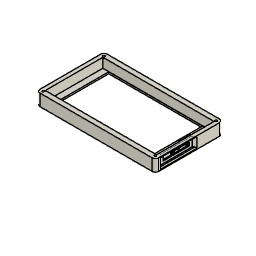
Display Mount - TFT70V30 SD Access Cover (Autodesk Fusion 360 design; units mm, degrees)
Autodesk Fusion 360 part; units mm, degrees
sketch "Sketch1" plane through (0, 0, -12) normal (0, 0, -1) x (1, 0, 0)
  line L0 (-106, 54.1) -> (-106, -54.1)
  line L1 (-100, -60.1) -> (100, -60.1)
  line L2 (106, -54.1) -> (106, 54.1)
  line L3 (100, 60.1) -> (-100, 60.1)
  arc A0 (4.9335, 51.1) -> (-4.9335, 51.1) centre (0, 51.9125) ccw
  arc A1 (86.5835, 51.1) -> (76.7165, 51.1) centre (81.65, 51.9125) ccw
  line L4 (86.5835, 51.1) -> (99, 51.1)
  line L5 (99, 51.1) -> (99, -51.1)
  line L6 (99, -51.1) -> (86.5835, -51.1)
  arc A2 (76.7165, -51.1) -> (86.5835, -51.1) centre (81.65, -51.9125) ccw
  arc A3 (-4.9335, -51.1) -> (4.9335, -51.1) centre (0, -51.9125) ccw
  arc A4 (-86.5835, -51.1) -> (-76.7165, -51.1) centre (-81.65, -51.9125) ccw
  line L7 (-86.5835, -51.1) -> (-99, -51.1)
  line L8 (-99, -51.1) -> (-99, 51.1)
  line L9 (-99, 51.1) -> (-86.5835, 51.1)
  arc A5 (-76.7165, 51.1) -> (-86.5835, 51.1) centre (-81.65, 51.9125) ccw
  circle A6 centre (-100, -54.1) radius 2.3
  circle A7 centre (100, -54.1) radius 2.3
  circle A8 centre (-100, 54.1) radius 2.3
  circle A9 centre (100, 54.1) radius 2.3
  arc A10 (106, 54.1) -> (100, 60.1) centre (100, 54.1) ccw
  arc A11 (-100, 60.1) -> (-106, 54.1) centre (-100, 54.1) ccw
  arc A12 (-106, -54.1) -> (-100, -60.1) centre (-100, -54.1) ccw
  arc A13 (100, -60.1) -> (106, -54.1) centre (100, -54.1) ccw
  line L10 (5.2198, 51.35) -> (76.4302, 51.35)
  line L11 (-5.2198, -51.35) -> (-76.4302, -51.35)
  line L12 (76.4302, -51.35) -> (5.2198, -51.35)
  line L13 (-86.5835, 51.1) -> (86.5835, 51.1)
  circle A14 centre (-100, 54.1) radius 1.925
  circle A15 centre (100, 54.1) radius 1.925
  circle A16 centre (-100, -54.1) radius 1.925
  circle A17 centre (100, -54.1) radius 1.925
  line L14 (-76.7165, 51.1) -> (-4.9335, 51.1)
  line L15 (4.9335, 51.1) -> (76.7165, 51.1)
  line L16 (76.7165, -51.1) -> (4.9335, -51.1)
  line L17 (-4.9335, -51.1) -> (-76.7165, -51.1)
  line L18 (-99.3, 51.4) -> (99.3, 51.4)
  line L19 (99.3, 51.4) -> (99.3, -51.4)
  line L20 (99.3, -51.4) -> (-99.3, -51.4)
  line L21 (-99.3, -51.4) -> (-99.3, 51.4)
  dimension "d90" = 3.85
  dimension "d91" = 3.85
  dimension "d96" = 3.85
  dimension "d97" = 3.85
  dimension "d105" = 0.3
  dimension "d106" = 0.3
  dimension "d107" = 0.3
  dimension "d108" = 0.3
  constraint coincident L9.end A5.end
  constraint coincident A1.start L4.start
  constraint concentric A8 A14
  constraint concentric A9 A15
  constraint concentric A6 A16
  constraint concentric A7 A17
  constraint horizontal L18
  constraint vertical L19
  constraint horizontal L20
  constraint vertical L21
  measures "d90" diameter of A14
  measures "d91" diameter of A15
  measures "d96" diameter of A16
  measures "d97" diameter of A17
  measures "d105" distance of L5 L19
  measures "d106" distance of L6 L20
  measures "d107" distance of L8 L21
  measures "d108" distance of L9 L18
extrude "Extrude2" add sketch "Sketch1" along normal blind 17 contours L0 L1 L2 L3 A10 A11 A12 A13 | A6 | A7 | A8 | A9
extrude "Extrude13" add sketch "Sketch1" along normal blind 17 contours A0 L18 | A1 L18 | A5 L18 | A2 L20 | A4 L20 | A3 L20
sketch "Sketch2" plane through (0, 0, -29) normal (0, 0, -1) x (1, 0, 0)
  circle A0 centre (-100, -54.1) radius 1.925
  circle A1 centre (100, 54.1) radius 1.925
  circle A2 centre (100, -54.1) radius 1.925
  line L0 (-99.3, -51.4) -> (-99.3, 51.4)
  line L1 (-99.3, 51.4) -> (99.3, 51.4)
  line L2 (99.3, 51.4) -> (99.3, -51.4)
  line L3 (99.3, -51.4) -> (-99.3, -51.4)
  circle A3 centre (-100, 54.1) radius 1.925
  arc A4 (100, -60.1) -> (106, -54.1) centre (100, -54.1) ccw
  line L4 (106, -54.1) -> (106, 54.1)
  arc A5 (106, 54.1) -> (100, 60.1) centre (100, 54.1) ccw
  line L5 (100, 60.1) -> (-100, 60.1)
  arc A6 (-100, 60.1) -> (-106, 54.1) centre (-100, 54.1) ccw
  line L6 (-106, 54.1) -> (-106, -54.1)
  arc A7 (-106, -54.1) -> (-100, -60.1) centre (-100, -54.1) ccw
  line L7 (-100, -60.1) -> (100, -60.1)
extrude "Extrude3" add sketch "Sketch2" along normal blind 4 contours A0 | A1 | A2 | L0 L1 L2 L3 | A3 | A4 L4 A5 L5 A6 L6 A7 L7
sketch "Sketch3" plane through (0, 0, -33) normal (0, 0, -1) x (1, 0, 0)
  line L0 (-100, -60.1) -> (100, -60.1)
  arc A0 (100, -60.1) -> (106, -54.1) centre (100, -54.1) ccw
  line L1 (106, -54.1) -> (106, 54.1)
  arc A1 (106, 54.1) -> (100, 60.1) centre (100, 54.1) ccw
  line L2 (100, 60.1) -> (-100, 60.1)
  arc A2 (-100, 60.1) -> (-106, 54.1) centre (-100, 54.1) ccw
  line L3 (-106, 54.1) -> (-106, -54.1)
  arc A3 (-106, -54.1) -> (-100, -60.1) centre (-100, -54.1) ccw
  line L4 (-144.4997, -1.2493) -> (144.4997, 1.2493) construction
  line L5 (0, 97.7484) -> (0, -97.7484) construction
  line L6 (-144.4997, -60.1) -> (144.4997, -60.1)
  circle A4 centre (89.25, -36.35) radius 2.2
  circle A5 centre (88, -16.85) radius 5
  line L7 (79.5, -6.85) -> (96.5, -6.85)
  line L8 (96.5, -6.85) -> (96.5, -26.85)
  line L9 (96.5, -26.85) -> (79.5, -26.85)
  line L10 (79.5, -26.85) -> (79.5, -6.85)
  line L11 (96.5, -6.85) -> (79.5, -26.85) construction
  circle A6 centre (89.5, 11.4) radius 1.5
  circle A7 centre (89.5, 11.4) radius 7.5
  line L12 (-88.6, 51.1) -> (79, 51.1)
  line L13 (79, 51.1) -> (79, -51.1)
  line L14 (79, -51.1) -> (-88.6, -51.1)
  line L15 (-88.6, -51.1) -> (-88.6, 51.1)
  line L16 (82.25, -29.35) -> (96.25, -29.35)
  line L17 (96.25, -29.35) -> (96.25, -43.35)
  line L18 (96.25, -43.35) -> (82.25, -43.35)
  line L19 (82.25, -43.35) -> (82.25, -29.35)
  line L20 (96.25, -29.35) -> (82.25, -43.35) construction
  point P0 (88, -16.85)
  point P1 (89.25, -36.35)
  dimension "d114" = 4.4
  dimension "d115" = 23.75
  dimension "d116" = 16.75
  dimension "d117" = 10
  dimension "d118" = 43.25
  dimension "d119" = 18
  dimension "d120" = 17
  dimension "d121" = 20
  dimension "d122" = 3
  dimension "d123" = 71.5
  dimension "d124" = 16.5
  dimension "d125" = 15
  dimension "d128" = 17.4
  dimension "d129" = 9
  dimension "d131" = 9.8
  dimension "d168" = 9
  dimension "d169" = 27
  dimension "d170" = 14
  dimension "d171" = 14
  constraint midpoint origin L4
  constraint perpendicular L0 L5
  constraint midpoint origin L5
  constraint perpendicular L5 L6
  constraint collinear L0 L6
  constraint horizontal L7
  constraint vertical L8
  constraint horizontal L9
  constraint vertical L10
  constraint midpoint L11 P0
  constraint coincident P0 A5.centre
  constraint concentric A6 A7
  constraint horizontal L12
  constraint vertical L13
  constraint horizontal L14
  constraint vertical L15
  constraint horizontal L16
  constraint vertical L17
  constraint horizontal L18
  constraint vertical L19
  constraint midpoint L20 P1
  constraint coincident P1 A4.centre
  measures "d114" diameter of A4
  measures "d115" distance of L6 P1
  measures "d116" distance of L1 P1
  measures "d117" diameter of A5
  measures "d118" distance of L6 P0
  measures "d119" distance of L1 P0
  measures "d120" distance of L7.start L7.end
  measures "d121" distance of L7.start L9.end
  measures "d122" diameter of A6
  measures "d123" distance of L6 A6.centre
  measures "d124" distance of L1 A6.centre
  measures "d125" diameter of A7
  measures "d128" distance of L3 L15
  measures "d129" distance of L2 L12
  measures "d168" distance of L6 L14
  measures "d169" distance of L1 L13
  measures "d170" distance of L16.start L16.end
  measures "d171" distance of L16.start L18.end
extrude "Extrude14" cut sketch "Sketch3" against normal blind 4 from surface at -1 contours L16 L17 L18 L19
extrude "Extrude5" cut sketch "Sketch3" against normal blind 3 from surface at -1 contours A7
extrude "Extrude4" cut sketch "Sketch3" against normal blind 4 contours L12 L13 L14 L15
extrude "Extrude6" cut sketch "Sketch3" against normal blind 4 contours A6
extrude "Extrude7" cut sketch "Sketch3" against normal blind 4 from surface at -0.8 contours L7 L8 L9 L10
extrude "Extrude8" cut sketch "Sketch3" against normal blind 4 contours A5
extrude "Extrude9" cut sketch "Sketch3" against normal blind 4 contours A4
sketch "Sketch4" plane through (106, 0, 0) normal (1, 0, 0) x (0, 1, 0)
  line L0 (54.1, -12) -> (-54.1, -12)
  line L1 (-54.1, -12) -> (-54.1, -33)
  line L2 (-54.1, -33) -> (54.1, -33)
  line L3 (54.1, -33) -> (54.1, -12)
  line L4 (5.1, -25.4) -> (-24.9, -25.4)
  line L5 (-24.9, -25.4) -> (-24.9, -19.4)
  line L6 (-24.9, -19.4) -> (5.1, -19.4)
  line L7 (5.1, -19.4) -> (5.1, -25.4)
  line L8 (-26.9, -25.4) -> (-41.7, -25.4)
  line L9 (-41.7, -25.4) -> (-41.7, -15.8)
  line L10 (-41.7, -15.8) -> (-26.9, -15.8)
  line L11 (-26.9, -15.8) -> (-26.9, -25.4)
  line L12 (60.1, -12) -> (60.1, -33)
  line L13 (-51.4, -12) -> (51.4, -12)
  line L14 (-46.7, -13.3) -> (10.1, -13.3)
  line L15 (10.1, -13.3) -> (10.1, -29.4)
  line L16 (10.1, -29.4) -> (-46.7, -29.4)
  line L17 (-46.7, -29.4) -> (-46.7, -13.3)
  dimension "d146" = 55
  dimension "d147" = 85
  dimension "d148" = 6
  dimension "d150" = 87
  dimension "d151" = 101.8
  dimension "d152" = 9.6
  dimension "d156" = 5
  dimension "d157" = 5
  dimension "d158" = 2.5
  dimension "d159" = 4
  dimension "d175" = 7.6
  constraint horizontal L4
  constraint vertical L5
  constraint horizontal L6
  constraint vertical L7
  constraint horizontal L8
  constraint vertical L9
  constraint horizontal L10
  constraint vertical L11
  constraint collinear L4 L8
  constraint horizontal L14
  constraint vertical L15
  constraint horizontal L16
  constraint vertical L17
  measures "d146" distance of L7 L12
  measures "d147" distance of L5 L12
  measures "d148" distance of L4 L6
  measures "d150" distance of L11 L12
  measures "d151" distance of L9 L12
  measures "d152" distance of L8 L10
  measures "d156" distance of L9 L17
  measures "d157" distance of L7 L15
  measures "d158" distance of L10 L14
  measures "d159" distance of L8 L16
  measures "d175" distance of L2 L4
extrude "Extrude12" cut sketch "Sketch4" against normal blind 4.5 contours L14 L15 L16 L17
extrude "Extrude10" cut sketch "Sketch4" against normal blind 6.7 contours L4 L5 L6 L7 | L8 L9 L10 L11
chamfer "Chamfer2" distance 4 angle 45 2 edges at (106, -46.7, -21.35) (106, 10.1, -21.35)
chamfer "Chamfer3" distance 2 angle 45 1 edges at (106, -18.3, -29.4)
chamfer "Chamfer4" distance 2 distance2 1 4 edges at (-4.8, -51.1, -33) (-88.6, 0, -33) (79, 0, -33) (-4.8, 51.1, -33) measured on face at (91.6545, -39.3422, -33) measured on face at (91.6545, -39.3422, -33) measured on face at (91.6545, -39.3422, -33) measured on face at (91.6545, -39.3422, -33)
equation "d91 = d90"
equation "d96 = d90"
equation "d97 = d90"
equation "d139 = 0 mm - 0.800 mm"
